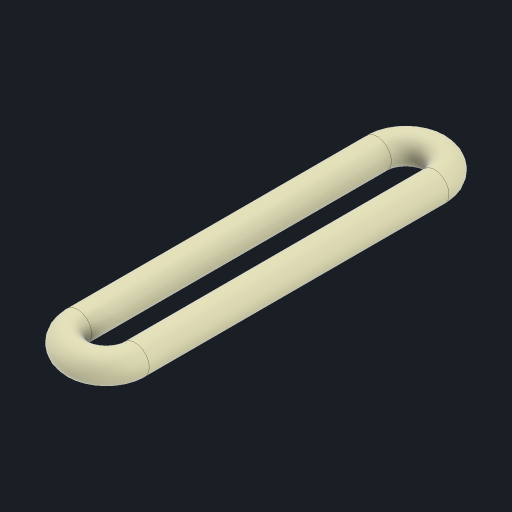
# Autodesk Inventor part: OUTK_011_Tubing
Saved by Autodesk Inventor 2024.2 (Build 282272000, 272)
## iProperties
Created: 2024-11-28
Part Number: OUTK_011_Tubing
Material: Rubber
Document SubType Name: Modeling
Designer: Bryan
Density: 0.93 g/cm^3
Appearance: Smooth - Ash
Author: Bryan
Autodesk Inventor part; units mm, degrees
ref_plane "YZ Plane" through (0, 0, 0) normal (1, 0, 0) x (0, 1, 0)
ref_plane "XZ Plane" through (0, 0, 0) normal (0, 1, 0) x (-1, 0, 0)
ref_plane "XY Plane" through (0, 0, 0) normal (0, 0, 1) x (1, 0, 0)
sketch "Sketch1" plane through (0, 0, 0) normal (0, 1, 0) x (-1, 0, 0)
  circle A0 centre (0, 0) radius 22.225 construction
  circle A1 centre (0, -231.2932) radius 22.225 construction
  line L0 (22.225, 0) -> (22.225, -231.2932)
  line L1 (-22.225, -231.2932) -> (-22.225, 0)
  arc A2 (22.225, 0) -> (-22.225, 0) centre (0, 0) ccw
  arc A3 (-22.225, -231.2932) -> (22.225, -231.2932) centre (0, -231.2932) ccw
  dimension "d0" = 44.45
  dimension "d1" = 231.2932
  constraints: 8 point on circle, 5 tangent, 4 centre point, 4 end point, 2 vertical, 1 coincident, 1 equal radius, 1 vertical alignment
  measures "d0" diameter of A0
  measures "d1" distance of point (0, 0) A1.centre
sketch "Sketch2" plane through (0, 0, 0) normal (0, 0, 1) x (1, 0, 0)
  line L0 (22.225, 0) -> (-22.225, 0) construction
  circle A0 centre (22.225, 0) radius 11.1125
  circle A1 centre (22.225, 0) radius 7.9375
  point P0 (0, 0)
  dimension "d2" = 22.225
  dimension "d3" = 3.175
  constraints: 2 centre point, 1 coincident
  measures "d2" diameter of A0
  measures "d3" radial gap between concentric circles of A0 A1
sweep "Sweep1" add profiles "Sketch2" path "Sketch1"
body "Solid1"
